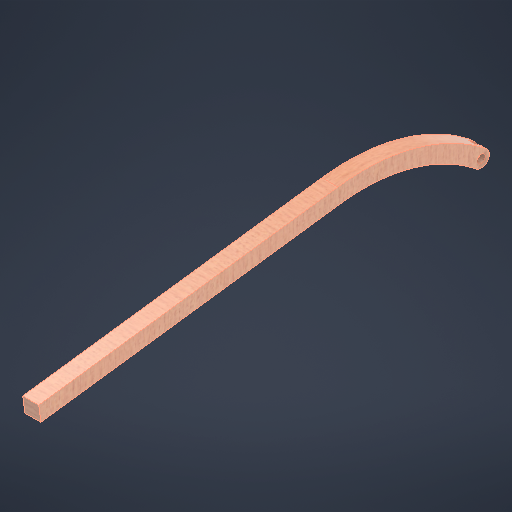
# Autodesk Inventor part: COUNTERWEIGHT_OUTSIDE_ARM,TREBUCHET
Saved by Autodesk Inventor 2026.2 (Build 302298010, 298A)
## iProperties
Created: 2026-02-12
Part Number: COUNTERWEIGHT_OUTSIDE_ARM,TREBUCHET
Material: Wood (Oak)
Document SubType Name: Modeling
Designer: 4aida
Density: 0.76 g/cm^3
Appearance: White Oak - Natural Medium Gloss
Author: 4aida
Autodesk Inventor part; units mm, degrees
ref_plane "YZ Plane" through (0, 0, 0) normal (1, 0, 0) x (0, 1, 0)
ref_plane "XZ Plane" through (0, 0, 0) normal (0, 1, 0) x (-1, 0, 0)
ref_plane "XY Plane" through (0, 0, 0) normal (0, 0, 1) x (1, 0, 0)
sketch "Sketch3" plane through (0, 0, 0) normal (1, 0, 0) x (0, 1, 0)
  line L0 (0, 700) -> (0, 0) construction
  circle A0 centre (0, 0) radius 6.35
  arc A1 (0, 0) -> (62.4484, 225.6573) centre (-234.9851, 186.4994) ccw construction
  line L1 (0, 700) -> (62.4484, 225.6573) construction
  arc A2 (-9.9477, 7.8951) -> (49.8571, 223.9996) centre (-234.9851, 186.4994) ccw
  line L2 (49.8571, 223.9996) -> (-12.5913, 698.3423)
  arc A3 (9.9477, -7.8951) -> (75.0398, 227.3149) centre (-234.9851, 186.4994) ccw
  line L3 (75.0398, 227.3149) -> (12.5913, 701.6577)
  arc A4 (-9.9477, 7.8951) -> (9.9477, -7.8951) centre (0, 0) ccw
  line L4 (-12.5913, 698.3423) -> (12.5913, 701.6577)
  dimension "d8" = 700
  dimension "d9" = 12.7
  dimension "d10" = 7.5
  dimension "d11" = 300
  dimension "d12" = 25.4
  dimension "d13" = 12.7
  constraints: 10 end point, 8 point on circle, 5 centre point, 2 coincident, 2 tangent, 1 midpoint, 1 perpendicular, 1 vertical, 2 other
  measures "d8" distance of L0.start L0.end
  measures "d9" diameter of A0
  measures "d10" angle of L1 L0
  measures "d11" radius of A1
  measures "d12" distance between parallel lines of L3 L2
  measures "d13" distance between parallel lines of L1 L2
extrude "Extrusion3" add sketch "Sketch3" along normal mid plane 25.4
sketch "Sketch4" plane through (0, 0, 0) normal (1, 0, 0) x (0, 1, 0)
  arc A0 (-9.9477, 7.8951) -> (9.9477, -7.8951) centre (0, 0) ccw projected
  circle A1 centre (0, 0) radius 12.7
  line L0 (17.9728, 2.6368) -> (-2.5885, 17.5818)
  arc A2 (-9.9477, 7.8951) -> (49.8571, 223.9996) centre (-234.9851, 186.4994) ccw projected
  arc A3 (9.9477, -7.8951) -> (75.0398, 227.3149) centre (-234.9851, 186.4994) ccw projected
  arc A4 (9.9477, -7.8951) -> (75.0398, 227.3149) centre (-234.9851, 186.4994) ccw projected
  point P0 (9.9477, -7.8951)
  point P1 (7.4669, 10.273)
  point P2 (9.9477, -7.8951)
  point P3 (17.9575, 2.6479)
  constraints: 2 end point, 1 coincident, 1 line through centre, 1 point on circle, 4 other
extrude "Extrusion4" cut sketch "Sketch4" along normal mid plane 9.525
equation "\"d13\" = 0.5 * d12"
body "Solid2"
